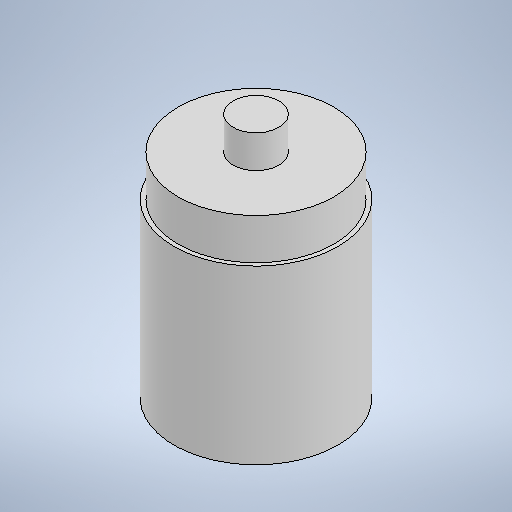
# Autodesk Inventor part: Pulse compensator
Saved by Autodesk Inventor 2025 (Build 290162010, 162A)
## iProperties
Created: 2025-06-03
Part Number: Pulse compensator
Material: Generic
Document SubType Name: Modeling
Designer: user
Density: 1 g/cm^3
Appearance: Default
Mass: 1008.23 g
Surface Area: 591.313 cm^2
Volume: 1008.23 cm^3
Author: user
Autodesk Inventor part; units mm, degrees
ref_plane "YZ Plane" through (0, 0, 0) normal (1, 0, 0) x (0, 1, 0)
ref_plane "XZ Plane" through (0, 0, 0) normal (0, 1, 0) x (-1, 0, 0)
ref_plane "XY Plane" through (0, 0, 0) normal (0, 0, 1) x (1, 0, 0)
sketch "Sketch1" plane through (0, 0, 0) normal (0, 1, 0) x (-1, 0, 0)
  line L0 (0, 0) -> (0, 150)
  line L1 (0, 150) -> (-14, 150)
  line L2 (-14, 150) -> (-14, 130)
  line L3 (-14, 130) -> (-47.5, 130)
  line L4 (-47.5, 130) -> (-47.5, 105)
  line L5 (-47.5, 105) -> (-50, 105)
  line L6 (-50, 105) -> (-50, 0)
  line L7 (-50, 0) -> (0, 0)
  dimension "d0" = 20
  dimension "d1" = 130
  dimension "d2" = 95
  dimension "d3" = 100
  dimension "d4" = 25
  dimension "d5" = 28
  constraints: 16 end point, 7 perpendicular, 1 vertical
  measures "d0" distance of L1.end L2.end
  measures "d1" distance between parallel lines of L7 L3
  measures "d2" diameter of L4 L0
  measures "d3" diameter of L6 L0
  measures "d4" distance of L3.end L4.end
  measures "d5" diameter of L2 L0
revolve "Revolution1" add sketch "Sketch1" angle 360 about axis through (0, 0, 0) along (0, 0, 1)
sketch "Sketch2" plane through (0, 0, 0) normal (0, 0, -1) x (-1, 0, 0)
  point P0 (0, 0)
hole "Hole1" at (0, 0, 0) direction (0, 0, 1) diameter 18.631 depth 20 tip angle 118 thread size "G20.955x1.814" designation "G 1/2" standard "ISO Pipe Threads"
body "Solid1"
